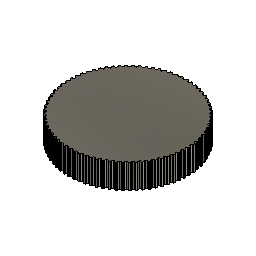
gear_78z (Autodesk Fusion 360 design; units mm, degrees)
Autodesk Fusion 360 part; units mm, degrees
sketch "Sketch1" plane through (0, 0, 0) normal (0, 0, 1) x (1, 0, 0) in component "gt2 pulley"
  circle A0 centre (0, 0) radius 24.8282 construction
  circle A1 centre (0, 0) radius 23.8242 construction
  line L0 (0, 0) -> (0, 24.8282) construction
  line L1 (0, 0) -> (0.9997, 24.808) construction
  line L2 (0, 0) -> (1.405, 24.7884) construction
  circle A2 centre (0, 0) radius 24.5742 construction
  arc A3 (0.3954, 24.4375) -> (0.4716, 24.1407) centre (1.3906, 24.5348) ccw
  circle A4 centre (0, 0) radius 24.4242 construction
  arc A5 (0.2475, 24.5729) -> (0, 24.5742) centre (0, 0) ccw
  arc A6 (0.3954, 24.4375) -> (0.2475, 24.5729) centre (0.2461, 24.4229) ccw
  arc A7 (0.4716, 24.1407) -> (0.9593, 23.8048) centre (0.9817, 24.3594) ccw
  arc A8 (0, 24.5742) -> (-0.2475, 24.5729) centre (0, 0) ccw
  arc A9 (-0.2475, 24.5729) -> (-0.3954, 24.4375) centre (-0.2461, 24.4229) ccw
  arc A10 (-0.4716, 24.1407) -> (-0.3954, 24.4375) centre (-1.3906, 24.5348) ccw
  arc A11 (-0.9594, 23.8048) -> (-0.4716, 24.1407) centre (-0.9817, 24.3594) ccw
  arc A12 (0.9593, 23.8048) -> (-0.9593, 23.8048) centre (0, 0) ccw
  point P0 (1.3906, 24.5348)
  point P1 (0, 24.5742)
  dimension "d18" = 49.6563
  dimension "d19" = 2.308
  dimension "d22" = 1.004
  dimension "d24" = 0.75
  dimension "d26" = 1
  dimension "d27" = 0.15
  dimension "d28" = 0.15
  dimension "d47" = 0.555
  dimension "d52" = 3.812
  constraint coincident A0.centre A1.centre
  constraint coincident A0 L0.end
  constraint vertical L0
  constraint coincident A0 L1.end
  constraint coincident A0 L2.end
  constraint concentric A1 A2
  constraint coincident A1 A7.end
  constraint coincident L1 A7.end
  constraint coincident A2 P0
  constraint coincident L2 P0
  constraint coincident P0 A3.centre
  constraint coincident A2 P1
  constraint coincident L0 P1
  constraint concentric A2 A4
  constraint coincident P1 A5.end
  constraint coincident A4 A6.centre
  constraint coincident A3.start A6.start
  constraint tangent A3 A6
  constraint tangent A3 A7
  constraint symmetric L0 A7.end A12.end
  constraint symmetric L0 A3.start A9.end
  constraint symmetric L0 A3.end A10.start
  constraint symmetric L0 A3 A10
  constraint symmetric L0 A5.start A8.end
  constraint symmetric L0 P1 A5.end
  constraint symmetric L0 A5 A8
  constraint symmetric L0 A6 A9
  constraint symmetric L0 A7 A11
  constraint coincident A1 A11.start
  constraint tangent A1 A7
  constraint coincident L1 A7.centre
  measures "d18" diameter of A0
  measures "d19" angle of L0 L1
  measures "d22" distance of A0 A1
  measures "d24" distance of A1 A2
  measures "d26" radius of A3
  measures "d27" distance of A2 A4
  measures "d28" radius of A6
  measures "d47" radius of A7
extrude "Extrude1" add sketch "Sketch1" along normal blind 10 makes body 1
pattern_circular "C-Pattern1" count 78 over 360 about axis through (0, 0, 1.75) along (0, 0, 1) of bodies 1 makes body 2 at (-1.1723, 23.7953, 3.3333) makes body 3 at (-3.0833, 23.6238, 6.6667) makes body 4 at (-5.598, 23.1572, 6.6667) makes body 5 at (-8.2485, 22.3507, 6.6667) makes body 6 at (-10.0203, 21.6145, 6.6667) makes body 7 at (-10.4055, 21.4317, 3.3333) makes body 8 at (-12.8232, 20.0787, 6.6667) makes body 9 at (-13.7086, 19.485, 3.3333) makes body 10 at (-15.878, 17.7617, 6.6667) makes body 11 at (-16.6567, 17.0336, 3.3333) makes body 12 at (-18.3867, 15.1499, 6.6667) makes body 13 at (-20.0212, 12.9129, 6.6667) makes body 14 at (-20.9954, 11.2599, 6.6667) makes body 15 at (-21.8333, 9.534, 6.6667) makes body 16 at (-22.3136, 8.3484, 6.6667) makes body 17 at (-22.6647, 7.3418, 3.3333) makes body 18 at (-23.3211, 4.8698, 6.6667) makes body 19 at (-23.5489, 3.611, 3.3333) makes body 20 at (-23.8089, 0.8527, 6.6667) makes body 21 at (-23.8232, -0.2132, 3.3333) makes body 22 at (-23.7288, -2.1295, 3.3333) makes body 23 at (-23.3211, -4.8699, 6.6667) makes body 24 at (-22.6647, -7.3419, 6.6667) makes body 25 at (-22.5297, -7.7463, 3.3333) makes body 26 at (-21.1935, -10.8825, 6.6667) makes body 27 at (-20.6854, -11.8197, 6.6667) makes body 28 at (-19.1734, -14.1412, 6.6667) makes body 29 at (-18.1125, -15.4767, 6.6667) makes body 30 at (-16.8085, -16.8839, 6.6667) makes body 31 at (-16.3491, -17.3291, 3.3333) makes body 32 at (-13.7086, -19.485, 6.6667) makes body 33 at (-12.6429, -20.1928, 6.6667) makes body 34 at (-11.7269, -20.7381, 3.3333) makes body 35 at (-8.6471, -22.1995, 6.6667) makes body 36 at (-8.2484, -22.3507, 3.3333) makes body 37 at (-5.5979, -23.1572, 6.6667) makes body 38 at (-4.5563, -23.3844, 6.6667) makes body 39 at (-1.8107, -23.7553, 6.6667) makes body 40 at (0.1067, -23.8239, 6.6667) makes body 41 at (1.1723, -23.7953, 3.3333) makes body 42 at (3.7164, -23.5325, 6.6667) makes body 43 at (5.598, -23.1572, 6.6667) makes body 44 at (8.2485, -22.3507, 6.6667) makes body 45 at (10.0203, -21.6145, 6.6667) makes body 46 at (10.4055, -21.4317, 3.3333) makes body 47 at (12.0963, -20.5249, 3.3333) makes body 48 at (13.7086, -19.485, 3.3333) makes body 49 at (15.878, -17.7617, 6.6667) makes body 50 at (17.2558, -16.4265, 6.6667) makes body 51 at (17.9733, -15.6381, 6.6667) makes body 52 at (20.0212, -12.9129, 6.6667) makes body 53 at (20.6855, -11.8196, 6.6667) makes body 54 at (21.8333, -9.534, 6.6667) makes body 55 at (22.3136, -8.3484, 6.6667) makes body 56 at (23.0799, -5.9082, 6.6667) makes body 57 at (23.3211, -4.8698, 6.6667) makes body 58 at (23.6631, -2.7658, 6.6667) makes body 59 at (23.8089, -0.8527, 6.6667) makes body 60 at (23.7631, 1.7045, 6.6667) makes body 61 at (23.7288, 2.1295, 3.3333) makes body 62 at (23.3211, 4.8699, 6.6667) makes body 63 at (22.8536, 6.7307, 6.6667) makes body 64 at (22.5297, 7.7463, 3.3333) makes body 65 at (21.8333, 9.5341, 3.3333) makes body 66 at (20.5788, 12.0043, 6.6667) makes body 67 at (19.1734, 14.1412, 6.6667) makes body 68 at (18.5215, 14.9848, 6.6667) makes body 69 at (17.108, 16.5803, 6.6667) makes body 70 at (16.3491, 17.3291, 3.3333) makes body 71 at (13.7086, 19.485, 6.6667) makes body 72 at (12.6429, 20.1928, 6.6667) makes body 73 at (11.7269, 20.7381, 3.3333) makes body 74 at (8.6471, 22.1995, 6.6667) makes body 75 at (8.2484, 22.3507, 3.3333) makes body 76 at (6.4232, 22.942, 3.3333) makes body 77 at (3.9268, 23.4983, 6.6667) makes body 78 at (1.8107, 23.7553, 6.6667)
sketch "Sketch2" plane through (0, 0, 10) normal (0, 0, 1) x (-1, 0, 0)
  arc A0 (-11.7068, -21.4546) -> (-11.6388, -21.6432) centre (-11.5678, -21.5111) ccw
  arc A1 (-11.6388, -21.6432) -> (-11.2004, -21.8733) centre (0, 0) ccw
  arc A2 (-11.2004, -21.8733) -> (-11.0066, -21.8221) centre (-11.132, -21.7398) ccw
  arc A3 (-10.8012, -21.5946) -> (-11.0066, -21.8221) centre (-10.1705, -22.3707) ccw
  arc A4 (-10.2132, -21.524) -> (-10.8012, -21.5946) centre (-10.4512, -22.0254) ccw
  arc A5 (-11.9121, -20.6323) -> (-10.2132, -21.524) centre (0, 0) ccw
  arc A6 (-11.6363, -21.1563) -> (-11.9121, -20.6323) centre (-12.1896, -21.113) ccw
  arc A7 (-11.7068, -21.4546) -> (-11.6363, -21.1563) centre (-12.6332, -21.0782) ccw
  circle A8 centre (0, 0) radius 23.8242
  constraint coincident A1.centre A5.centre
extrude "Extrude2" add sketch "Sketch2" against normal blind 10 contours A5 A8 bodies 1 2 3 4 5 6 7 8 9 10 11 12 13 14 15 16 17 18 19 20 21 22 23 24 25 26 27 28 29 30 31 32 33 34 35 36 37 38 39 40 41 42 43 44 45 46 47 48 49 50 51 52 53 54 55 56 57 58 59 60 61 62 63 64 65 66 67 68 69 70 71 72 73 74 75 76 77 78
extrude "Extrude4" [suppressed] in component "gt2 pulley"
pattern_circular "C-Pattern7" [suppressed] in component "gt2 pulley"
extrude "Extrude3" [suppressed] in component "gt2 pulley"
pattern_circular "C-Pattern6" [suppressed] in component "gt2 pulley"
extrude "Extrude2'" [suppressed] in component "gt2 pulley"
pattern_circular "C-Pattern5" [suppressed] in component "gt2 pulley"
extrude "Extrude1'" [suppressed] in component "gt2 pulley"
pattern_circular "C-Pattern4" [suppressed] in component "gt2 pulley"
pattern_circular "C-Pattern3" [suppressed] in component "gt2 pulley"
pattern_circular "C-Pattern2" [suppressed] in component "gt2 pulley"
pattern_circular "C-Pattern1'" [suppressed] in component "gt2 pulley"
copy_body "Body->Comp1" [suppressed] in component "Component"
copy_body "Body->Comp2" [suppressed] in component "Component'"
copy_body "Body->Comp3" [suppressed] in component "Component''"
copy_body "Body->Comp4" [suppressed] in component "Component'''"
copy_body "Body->Comp5" [suppressed] in component "Component''''"
copy_body "Body->Comp6" [suppressed] in component "Component'''''"
copy_body "Body->Comp7" [suppressed] in component "Component''''''"
copy_body "Body->Comp8" [suppressed] in component "Component'''''''"
copy_body "Body->Comp9" [suppressed] in component "Component''''''''"
copy_body "Body->Comp10" [suppressed] in component "Component'''''''''"
copy_body "Body->Comp11" [suppressed] in component "Component''''''''''"
copy_body "Body->Comp12" [suppressed] in component "Component'''''''''''"
copy_body "Body->Comp13" [suppressed] in component "Component''''''''''''"
copy_body "Body->Comp14" [suppressed] in component "Component'''''''''''''"
copy_body "Body->Comp15" [suppressed] in component "Component''''''''''''''"
copy_body "Body->Comp16" [suppressed] in component "Component'''''''''''''''"
copy_body "Body->Comp17" [suppressed] in component "Component''''''''''''''''"
copy_body "Body->Comp18" [suppressed] in component "Component'''''''''''''''''"
copy_body "Body->Comp19" [suppressed] in component "Component''''''''''''''''''"
copy_body "Body->Comp20" [suppressed] in component "Component'''''''''''''''''''"
component "gt2 pulley" placed x (1, 0, 0) y (0, 1, 0) z (0, 0, 1) at (0, 0, 0)
equation "NumTeeth = 78" comment "min 20"
equation "ToothPitch = 2 mm"
equation "PullyDia = NumTeeth * ToothPitch / PI"
equation "ToothAng = ( ( 360 / NumTeeth ) * 1 deg )"
equation "TransOffsetAngle = ToothAng * 0.2"
equation "Sholulder_Radius = 0.15 mm"
equation "Root_Radius = 0.555 mm"
equation "TransRadius = 1 mm"
equation "ToolHeight = 0.75 mm"
equation "PLD = 0.254 mm"
equation "d18 = PullyDia"
equation "d19 = ToothAng / 2"
equation "d22 = PLD + ToolHeight"
equation "d24 = ToolHeight"
equation "d26 = TransRadius"
equation "d27 = Sholulder_Radius"
equation "d31 = NumTeeth"
equation "d33 = NumTeeth"
equation "d35 = NumTeeth"
equation "d37 = NumTeeth"
equation "d41 = NumTeeth"
equation "d45 = NumTeeth"
equation "d47 = Root_Radius"
equation "d50 = NumTeeth"
